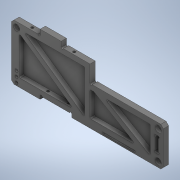
# Autodesk Inventor part: Cockpit_vertical_frame_03
Saved by Autodesk Inventor 2020.4 (Build 244396000, 396)
## iProperties
Created: 2021-04-12
Part Number: Cockpit_vertical_frame_03
Material: アセタール樹脂、黒
Document SubType Name: Modeling
Designer: Masato Kubotera
Density: 1.425 g/cm^3
Appearance: 滑らか - 黒
Mass: 26.6371 g
Surface Area: 177.414 cm^2
Volume: 18.6927 cm^3
Description: POM T5
d0: 145.000 mm
d1: 53.000 mm
d2: 75.000 mm
d3: 16.000 mm
d4: 2.500 mm
d5: 3.100 mm
d6: 2.500 mm
d7: 5.000 mm
d12: 20.000 mm
d13: 27.500 mm
d14: 5.000 mm
d15: 1.050 mm
d16: 1.050 mm
d53: 1.050 mm
d54: 1.050 mm
d55: 1.050 mm
d56: 1.050 mm
d59: 5.000 mm
d60: 0.00 deg
d107: 30.000 mm
d108: 1.500 mm
d109: 0.050 mm
d110: 0.050 mm
d114: 0.050 mm
d115: 0.050 mm
d116: 30.000 mm
d118: 5.000 mm
d120: 132.500 mm
d123: 2.500 mm
d124: 15.000 mm
d125: 0.050 mm
d126: 0.050 mm
d127: 1.050 mm
d128: 1.050 mm
d129: 1.050 mm
d130: 1.050 mm
d132: 30.000 mm
d134: 3.000 mm
d135: 2.500 mm
d140: 5.000 mm
d144: 5.000 mm
d146: 5.000 mm
d147: 20.000 mm
d152: 1.050 mm
d169: 6.000 mm
d170: 2.000 mm
d171: 0.00 deg
d172: 2.500 mm
d176: 20.000 mm
d177: 40.000 mm
d179: 5.000 mm
d183: 5.000 mm
d185: 5.000 mm
d186: 5.000 mm
d187: 5.000 mm
d188: 2.500 mm
d190: 8.000 mm
d191: 5.000 mm
d192: 5.000 mm
d193: 5.000 mm
d195: 5.000 mm
d196: 2.500 mm
d197: 1.000 mm
d198: 0.500 mm
d199: 0.00 deg
d17: 70.000 mm
d74: 37.000 mm
d133: 20.000 mm
d148: 130.000 mm
Author: Masato Kubotera
Title: Cockpit_vertical_frame_03
Autodesk Inventor part; units mm, degrees
ref_plane "YZ Plane" through (0, 0, 0) normal (1, 0, 0) x (0, 1, 0)
ref_plane "XZ Plane" through (0, 0, 0) normal (0, 1, 0) x (-1, 0, 0)
ref_plane "XY Plane" through (0, 0, 0) normal (0, 0, 1) x (1, 0, 0)
sketch "スケッチ2" plane through (-42.95, -23.5, 0) normal (0, -1, 0) x (1, 0, 0)
  line L0 (0, 0) -> (25.9, 5) construction
  line L1 (0, 5) -> (25.9, 5) projected
  line L2 (12.95, 5) -> (12.95, 0) construction
  line L3 (0, 0) -> (25.9, 0) projected
  line L4 (0, 0) -> (0, 5) projected
  line L5 (0, 2.5) -> (25.9, 2.5) construction
  line L6 (25.9, 0) -> (25.9, 5) projected
  point P0 (42.95, 0)
  point P1 (2.95, 2.5)
  point P2 (22.95, 2.5)
  dimension "d176" = 20
  constraints: 6 end point, 4 midpoint, 1 coincident, 1 point on line, 1 symmetric about line
  measures "d176" distance of point (22.95, 2.5) point (2.95, 2.5)
sketch "スケッチ1" plane through (0, 0, 0) normal (0, 0, 1) x (1, 0, 0)
  line L0 (-72.5, 26.5) -> (-47.1, 26.5)
  line L1 (72.5, 26.5) -> (72.5, 10.5) construction
  line L2 (-72.5, -26.5) -> (-72.5, 26.5)
  line L3 (-72.5, 26.5) -> (72.5, -26.5) construction
  line L4 (72.5, 26.5) -> (-72.5, -26.5) construction
  line L5 (2.5, 26.5) -> (2.5, 10.5)
  line L6 (2.5, 10.5) -> (4.6, 10.5) construction
  line L7 (2.5, 26.5) -> (72.5, 26.5) construction
  line L8 (72.5, 10.5) -> (72.5, -26.5)
  line L9 (70, 10.5) -> (70, -26) construction
  circle A0 centre (67.5, 5.5) radius 1.55
  line L10 (-45, 26.5) -> (-45, 31.5)
  line L11 (-45, 31.5) -> (-25, 31.5)
  line L12 (-25, 31.5) -> (-25, 26.5)
  line L13 (-45, 26.5) -> (-25, 26.5) construction
  line L14 (-25, 26.5) -> (-22.9, 26.5) construction
  arc A1 (-47.1, 26.5) -> (-45, 26.5) centre (-46.05, 26.5) ccw
  arc A2 (-25, 26.5) -> (-22.9, 26.5) centre (-23.95, 26.5) ccw
  line L15 (-47.1, 26.5) -> (-45, 26.5) construction
  line L16 (-22.9, 26.5) -> (2.5, 26.5)
  line L17 (65, 10.5) -> (65, -26.5) construction
  line L18 (-45.05, -23.5) -> (-42.95, -23.5) construction
  arc A3 (-42.95, -23.5) -> (-45.05, -23.5) centre (-44, -23.5) ccw
  arc A4 (-14.95, -23.5) -> (-17.05, -23.5) centre (-16, -23.5) ccw
  line L19 (-42.95, -23.5) -> (-17.05, -23.5)
  line L20 (-17.05, -23.5) -> (-14.95, -23.5) construction
  line L21 (15, -23.5) -> (45, -23.5) construction
  line L22 (45, -23.5) -> (45, -25) construction
  line L23 (45, -25) -> (15, -25) construction
  line L24 (15, -25) -> (15, -23.5) construction
  line L25 (15, -23.5) -> (45, -25) construction
  line L26 (45, -23.5) -> (15, -25) construction
  line L27 (14.95, -23.45) -> (45.05, -23.45)
  line L28 (45.05, -23.45) -> (45.05, -25.05) construction
  line L29 (45.05, -25.05) -> (14.95, -25.05)
  line L30 (14.95, -25.05) -> (14.95, -23.45) construction
  line L31 (14.95, -23.45) -> (45.05, -25.05) construction
  line L32 (45.05, -23.45) -> (14.95, -25.05) construction
  line L33 (-45, -23.5) -> (-45, -26.5) construction
  line L34 (-15, -23.5) -> (-15, -26.5) construction
  line L35 (72.5, -8) -> (-72.5, -8) construction
  line L36 (67.5, -0.5) -> (65, -0.5) construction
  line L37 (65, -0.5) -> (65, -15.5) construction
  line L38 (65, -15.5) -> (67.5, -15.5) construction
  line L39 (67.5, -15.5) -> (67.5, -0.5) construction
  line L40 (67.5, -0.5) -> (65, -15.5) construction
  line L41 (65, -0.5) -> (67.5, -15.5) construction
  line L42 (64.95, -0.45) -> (67.55, -0.45)
  line L43 (67.55, -0.45) -> (67.55, -2.55) construction
  line L44 (67.55, -15.55) -> (64.95, -15.55)
  line L45 (64.95, -15.55) -> (64.95, -13.45) construction
  line L46 (64.95, -0.45) -> (67.55, -15.55) construction
  line L47 (67.55, -0.45) -> (64.95, -15.55) construction
  arc A5 (64.95, -0.45) -> (64.95, -2.55) centre (64.95, -1.5) ccw
  arc A6 (67.55, -2.55) -> (67.55, -0.45) centre (67.55, -1.5) ccw
  arc A7 (64.95, -13.45) -> (64.95, -15.55) centre (64.95, -14.5) ccw
  arc A8 (67.55, -15.55) -> (67.55, -13.45) centre (67.55, -14.5) ccw
  line L48 (64.95, -2.55) -> (64.95, -0.45) construction
  line L49 (64.95, -13.45) -> (64.95, -2.55)
  line L50 (67.55, -13.45) -> (67.55, -15.55) construction
  line L51 (67.55, -2.55) -> (67.55, -13.45)
  arc A9 (14.95, -23.45) -> (14.95, -25.05) centre (14.95, -24.25) ccw
  arc A10 (45.05, -25.05) -> (45.05, -23.45) centre (45.05, -24.25) ccw
  circle A11 centre (67.5, -21.5) radius 1.55
  line L52 (-72.5, -26.5) -> (-45, -26.5)
  line L53 (-15, -26.5) -> (72.5, -26.5)
  line L54 (-45, -26.5) -> (-15, -26.5) construction
  line L55 (-70, 26) -> (-70, -26.5) construction
  line L56 (-65, 26.5) -> (-65, -26.5) construction
  arc A12 (2.5, 10.5) -> (4.6, 10.5) centre (3.55, 10.5) ccw
  line L57 (4.6, 10.5) -> (72.5, 10.5)
  circle A13 centre (67.5, 5.5) radius 3
  circle A14 centre (67.5, -21.5) radius 3
  line L58 (2.5, 5.5) -> (2.5, -18.5)
  line L59 (2.5, -18.5) -> (46.579, -18.5)
  line L60 (46.579, -18.5) -> (6.0385, 5.5)
  line L61 (15.8534, 5.5) -> (60, 5.5)
  line L62 (60, 5.5) -> (60, -20.6348)
  line L63 (60, -20.6348) -> (15.8534, 5.5)
  line L64 (-65, 18.1388) -> (-65, -18.5)
  line L65 (-65, -18.5) -> (-13.1527, -18.5)
  line L66 (-13.1527, -18.5) -> (-65, 18.1388)
  line L67 (-61.0926, 21.5) -> (-2.5, 21.5)
  line L68 (-2.5, 21.5) -> (-2.5, -19.9054)
  line L69 (-2.5, -19.9054) -> (-61.0926, 21.5)
  line L70 (-72.5, 26.5) -> (2.5, -26.5) construction
  line L71 (2.5, 10.5) -> (2.5, -26.5) construction
  line L72 (6.0385, 5.5) -> (2.5, 5.5)
  line L73 (2.5, 10.5) -> (65, -26.5) construction
  circle A15 centre (-67.5, 21.5) radius 1.25
  circle A16 centre (-67.5, 21.5) radius 3
  circle A17 centre (-67.5, -24) radius 1.5
  circle A18 centre (-67.5, -19) radius 1.5
  circle A19 centre (-67.5, -14) radius 1.5
  line L74 (-67.5, 26.5) -> (-67.5, -26.5) construction
  line L75 (-45.05, -23.5) -> (-45.05, -26.5)
  line L76 (-14.95, -23.5) -> (-14.95, -26.5)
  point P0 (0, 0)
  point P1 (30, -24.25)
  point P2 (66.25, -8)
  dimension "d0" = 145
  dimension "d1" = 53
  dimension "d2" = 75
  dimension "d3" = 16
  dimension "d4" = 2.5
  dimension "d5" = 3.1
  dimension "d6" = 2.5
  dimension "d7" = 5
  dimension "d12" = 20
  dimension "d13" = 27.5
  dimension "d14" = 5
  dimension "d15" = 1.05
  dimension "d16" = 1.05
  dimension "d17" = 70
  dimension "d55" = 1.05
  dimension "d56" = 1.05
  dimension "d74" = 37
  dimension "d107" = 30
  dimension "d108" = 1.5
  dimension "d109" = 0.05
  dimension "d110" = 0.05
  dimension "d116" = 30
  dimension "d118" = 5
  dimension "d123" = 2.5
  dimension "d124" = 15
  dimension "d125" = 0.05
  dimension "d126" = 0.05
  dimension "d127" = 1.05
  dimension "d128" = 1.05
  dimension "d129" = 1.05
  dimension "d130" = 1.05
  dimension "d132" = 30
  dimension "d133" = 20
  dimension "d134" = 3
  dimension "d135" = 2.5
  dimension "d146" = 5
  dimension "d147" = 20
  dimension "d148" = 130
  dimension "d152" = 1.05
  dimension "d169" = 6
  dimension "d185" = 5
  dimension "d186" = 5
  dimension "d187" = 5
  dimension "d188" = 2.5
  dimension "d190" = 8
  dimension "d191" = 5
  dimension "d192" = 5
  dimension "d193" = 5
  dimension "d195" = 5
  dimension "d196" = 2.5
  dimension "d200" = 2.5
  dimension "d201" = 6
  dimension "d204" = 5
  dimension "d205" = 2.5
  dimension "d206" = 3
  dimension "d207" = 3
  dimension "d208" = 3
  dimension "d209" = 2.5
  dimension "d210" = 2.5
  dimension "d211" = 5
  dimension "d212" = 5
  dimension "d213" = 0.05
  dimension "d214" = 0.05
  constraints: 154 end point, 39 perpendicular, 29 point on line, 22 midpoint, 22 point on circle, 21 parallel, 20 centre point, 18 horizontal, 5 vertical, 4 collinear, 2 coincident, 2 symmetric about line, 2 other
  measures "d0" distance of L3.end L2.start
  measures "d1" distance of L1.start L3.end
  measures "d2" distance between parallel lines of L2 L5
  measures "d3" distance of L5.start L5.end
  measures "d4" distance between parallel lines of L8 L9
  measures "d5" diameter of A0
  measures "d6" distance from line of L9 A0.centre
  measures "d7" distance from line of L6 A0.centre
  measures "d12" distance of L10.end L11.end
  measures "d13" distance between parallel lines of L2 L10
  measures "d14" distance between parallel lines of L11 L0
  measures "d15" radius of A1
  measures "d16" radius of A2
  measures "d17" distance of L5.end L1.end
  measures "d55" radius of A3
  measures "d56" radius of A4
  measures "d74" distance of L1.end L3.end
  measures "d107" distance of L22.end L23.end
  measures "d108" distance of L21.end L22.end
  measures "d109" distance between parallel lines of L30 L24
  measures "d110" distance between parallel lines of L27 L21
  measures "d116" distance between parallel lines of L33 L34
  measures "d118" distance between parallel lines of L9 L17
  measures "d123" distance of L37.end L38.end
  measures "d124" distance of L38.end L36.start
  measures "d125" distance between parallel lines of L42 L36
  measures "d126" distance between parallel lines of L43 L39
  measures "d127" radius of A5
  measures "d128" radius of A6
  measures "d129" radius of A8
  measures "d130" radius of A7
  measures "d132" distance between parallel lines of L24 L34
  measures "d133" distance between parallel lines of L17 L22
  measures "d134" distance between parallel lines of L52 L19
  measures "d135" distance between parallel lines of L2 L55
  measures "d146" distance between parallel lines of L55 L56
  measures "d147" distance between parallel lines of L56 L33
  measures "d148" distance between parallel lines of L17 L56
  measures "d152" radius of A12
  measures "d169" diameter of A13
  measures "d185" distance between parallel lines of L67 L13
  measures "d186" distance between parallel lines of L5 L68
  measures "d187" distance between parallel lines of L69 L66
  measures "d188" distance between parallel lines of L70 L66
  measures "d190" distance between parallel lines of L52 L65
  measures "d191" distance between parallel lines of L64 L55
  measures "d192" distance between parallel lines of L60 L63
  measures "d193" distance between parallel lines of L57 L61
  measures "d195" distance between parallel lines of L62 L17
  measures "d196" distance between parallel lines of L60 L73
  measures "d200" diameter of A15
  measures "d201" diameter of A16
  measures "d204" horizontal distance of L0.start A15.centre
  measures "d205" horizontal distance of A15.centre L55.start
  measures "d206" diameter of A17
  measures "d207" diameter of A18
  measures "d208" diameter of A19
  measures "d209" distance of L74.end L55.end
  measures "d210" distance of L74.end A17.centre
  measures "d211" distance of A17.centre A18.centre
  measures "d212" distance of A18.centre A19.centre
  measures "d213" distance between parallel lines of L75 L33
  measures "d214" distance between parallel lines of L76 L34
extrude "押し出し1" add sketch "スケッチ1" along normal blind 5 contours L0 A1 L10 L11 L12 A2 L16 L5 A12 L57 L8 L53 L76 A4 L19 A3 L75 L52 L2
extrude "押し出し2" add sketch "スケッチ1" along normal blind 2 contours A13 | A14 | A16
hole "穴1" at (-40, -23.5, 2.5) at (-20, -23.5, 2.5) direction (0, 1, 0) diameter 2.459 depth 5 thread size "M3x0.5" class "6H" standard "ISO Metric profile"
chamfer "面取り1" distance 2.5 angle 45 4 edges at (72.5, -26.5, 2.5) (72.5, 10.5, 2.5) (-72.5, 26.5, 2.5) (-72.5, -26.5, 2.5)
sketch "スケッチ3" plane through (-47.1, 26.5, 5) normal (0, 1, 0) x (1, 0, 0)
  line L0 (22.1, 0) -> (2.1, 0) projected
  line L1 (12.1, 0) -> (12.1, 5) construction
  line L2 (22.1, 5) -> (2.1, 5) projected
  line L3 (-22.9, 0) -> (-22.9, 5) projected
  line L4 (-22.9, 2.5) -> (49.6, 2.5) construction
  line L5 (49.6, 5) -> (49.6, 0) projected
  point P0 (47.1, 5)
  point P1 (-7.9, 2.5)
  point P2 (32.1, 2.5)
  dimension "d177" = 40
  constraints: 4 end point, 4 midpoint, 1 point on line, 1 symmetric about line
  measures "d177" distance of point (32.1, 2.5) point (-7.9, 2.5)
hole "穴2" at (-55, 26.5, 2.5) at (-15, 26.5, 2.5) direction (0, -1, 0) diameter 2.459 depth 5 thread size "M3x0.5" class "6H" standard "ISO Metric profile"
fillet "フィレット2" radius 1 13 edges at (-65, 18.1388, 2.5) (-61.0926, 21.5, 2.5) (-2.5, 21.5, 2.5) (-65, -18.5, 2.5) (-13.1527, -18.5, 2.5) (-2.5, -19.9054, 2.5) (2.5, -18.5, 2.5) (2.5, 5.5, 2.5) (6.0385, 5.5, 2.5) (15.8534, 5.5, 2.5) (60, 5.5, 2.5) (60, -20.6348, 2.5) (46.579, -18.5, 2.5)
extrude "押し出し4" add sketch "スケッチ1" along normal blind 0.5 contours L72 L60 L59 L58 | L61 L62 L63 | L66 L65 L64 | L67 L68 L69
equation "\"d13\" = -0.5 * d12 + 0.5 * d2"
equation "\"d16\" = d15"
equation "\"d55\" = d54"
equation "\"d56\" = d55"
equation "\"d53\" = d15"
equation "\"d54\" = d53"
